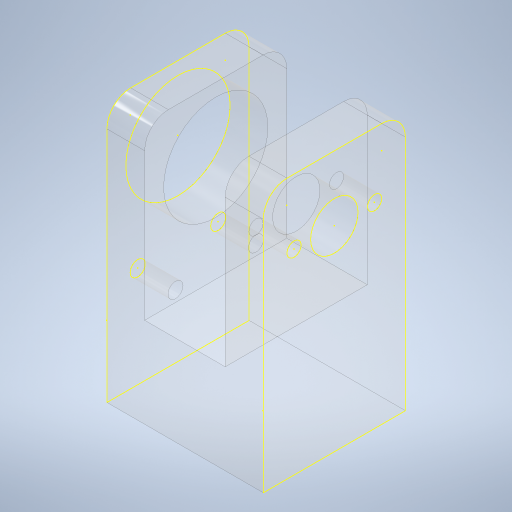
# Autodesk Inventor part: base
Saved by Autodesk Inventor 2024 (Build 280153000, 153)
## iProperties
Created: 2024-08-05
Part Number: base
Material: Polycarbonate, Clear
Document SubType Name: Modeling
Designer: David Ricaurte
Density: 1.2 g/cm^3
Appearance: Polycarbonate - Clear
Mass: 38.4086 g
Surface Area: 98.7251 cm^2
Volume: 32.0072 cm^3
Author: David Ricaurte
Autodesk Inventor part; units mm, degrees
ref_plane "YZ Plane" through (0, 0, 0) normal (1, 0, 0) x (0, 1, 0)
ref_plane "XZ Plane" through (0, 0, 0) normal (0, 1, 0) x (-1, 0, 0)
ref_plane "XY Plane" through (0, 0, 0) normal (0, 0, 1) x (1, 0, 0)
sketch "Sketch1" plane through (0, 0, 0) normal (1, 0, 0) x (0, 1, 0)
  line L0 (0, 0) -> (40, 0)
  line L1 (40, 0) -> (40, -30)
  line L2 (40, -30) -> (0, -30)
  line L3 (0, -30) -> (0, 0)
  line L4 (0, -15) -> (26.2886, -15)
  circle A0 centre (26.2886, -15) radius 8.5
  circle A1 centre (26.2886, -23.5) radius 1.5
  circle A2 centre (26.2886, -6.5) radius 1.5
  circle A3 centre (26.2886, -15) radius 5
  dimension "d0" = 40
  dimension "d1" = 30
  dimension "d2" = 17
  dimension "d3" = 3
  dimension "d4" = 3
  dimension "d5" = 10
  constraints: 10 end point, 4 centre point, 2 coincident, 2 horizontal, 2 parallel, 2 point on circle, 1 midpoint, 1 perpendicular
  measures "d0" distance of L1.end L2.end
  measures "d1" distance of L0.end L1.end
  measures "d2" diameter of A0
  measures "d3" diameter of A1
  measures "d4" diameter of A2
  measures "d5" diameter of A3
extrude "Extrusion1" add sketch "Sketch1" along normal blind 8 contours A0 A2 A1 | L0 L1 L2 L3
sketch "Sketch2" plane through (0, 0, 0) normal (-1, 0, 0) x (0, 0, 1)
  line L0 (0, 40) -> (0, 0) projected
  line L1 (-30, 0) -> (-30, 40) projected
  line L2 (0, 0) -> (-30, 0)
  line L3 (-30, 0) -> (-30, 4)
  line L4 (-30, 4) -> (0, 4)
  line L5 (0, 4) -> (0, 0)
  dimension "d8" = 4
  constraints: 8 end point, 2 parallel, 1 horizontal, 1 perpendicular, 1 point on line
  measures "d8" distance of L2.end L3.end
extrude "Extrusion2" add sketch "Sketch2" along normal blind 17
sketch "Sketch3" plane through (-17, 0, 0) normal (-1, 0, 0) x (0, 0, 1)
  line L0 (0, 40) -> (0, 0) projected
  line L1 (-30, 40) -> (0, 40) projected
  line L2 (0, 0) -> (-30, 0)
  line L3 (-30, 0) -> (-30, 40)
  line L4 (-30, 40) -> (0, 40)
  line L5 (0, 40) -> (0, 0)
  constraints: 8 end point, 2 parallel, 1 horizontal, 1 perpendicular
extrude "Extrusion3" add sketch "Sketch3" along normal blind 8
sketch "Sketch4" plane through (-17, 0, 0) normal (1, 0, 0) x (0, 0, -1)
  circle A0 centre (15, 26.2886) radius 5 projected
  circle A1 centre (15, 26.2886) radius 11
  point P0 (0, 0)
  dimension "d13" = 22
  constraints: 1 centre point, 1 coincident
  measures "d13" diameter of A1
extrude "Extrusion4" cut sketch "Sketch4" against normal through all contours A0 | A1
fillet "Fillet1" radius 5 4 edges at (4, 40, 0) (-21, 40, 0) (-21, 40, -30) (4, 40, -30)
sketch "Sketch5" plane through (-25, 0, 0) normal (-1, 0, 0) x (0, 0, 1)
  circle A0 centre (-15, 26.2886) radius 11 projected
  line L0 (-15, 26.2886) -> (-15, 6.2886)
  line L1 (-15, 6.2886) -> (-6.5, 6.2886)
  line L2 (-30, 35) -> (-30, 4) projected
  line L3 (-6.5, 6.2886) -> (-23.5, 6.2886)
  circle A1 centre (-6.5, 6.2886) radius 1.6
  circle A2 centre (-23.5, 6.2886) radius 1.6
  point P0 (0, 0)
  dimension "d17" = 20
  dimension "d18" = 8.5
  dimension "d19" = 17
  dimension "d20" = 3.2
  dimension "d21" = 3.2
  constraints: 6 end point, 2 centre point, 2 coincident, 1 perpendicular, 1 point on line, 1 vertical
  measures "d17" distance of L0.start L0.end
  measures "d18" distance of L0.end L1.end
  measures "d19" distance of L1.end L3.end
  measures "d20" diameter of A1
  measures "d21" diameter of A2
extrude "Extrusion5" cut sketch "Sketch5" against normal blind 10 contours A1 | A2
sketch "Sketch6" plane through (-25, 0, 0) normal (-1, 0, 0) x (0, 0, 1)
  line L0 (-30, 0) -> (-30, 35) projected
  line L1 (-30, 0) -> (0, 0)
  line L2 (0, 0) -> (0, -15)
  line L3 (0, -15) -> (-30, -15)
  line L4 (-30, -15) -> (-30, 0)
  dimension "d24" = 15
  constraints: 8 end point, 2 parallel, 1 horizontal, 1 perpendicular
  measures "d24" distance of L1.end L2.end
extrude "Extrusion6" add sketch "Sketch6" against normal blind 33
sketch "Sketch7" plane through (8, 0, 0) normal (1, 0, 0) x (0, 0, -1)
  arc A0 (30, 35) -> (25, 40) centre (25, 35) ccw projected
  line L0 (25, 40) -> (5, 40) projected
  arc A1 (5, 40) -> (0, 35) centre (5, 35) ccw projected
  line L1 (0, 35) -> (0, -15) projected
  line L2 (0, -15) -> (30, -15) projected
  line L3 (30, -15) -> (30, 35) projected
  circle A2 centre (23.5, 26.2886) radius 1.5 projected
  circle A3 centre (6.5, 26.2886) radius 1.5 projected
  circle A4 centre (15, 26.2886) radius 5 projected
  point P0 (0, 0)
sketch "Sketch8" plane through (-25, 0, 0) normal (-1, 0, 0) x (0, 0, 1)
  circle A0 centre (-23.5, 6.2886) radius 1.6 projected
  circle A1 centre (-6.5, 6.2886) radius 1.6 projected
  circle A2 centre (-15, 26.2886) radius 11 projected
  arc A3 (-25, 40) -> (-30, 35) centre (-25, 35) ccw projected
  line L0 (-30, 35) -> (-30, -15) projected
  line L1 (-30, -15) -> (0, -15) projected
  line L2 (0, -15) -> (0, 35) projected
  arc A4 (0, 35) -> (-5, 40) centre (-5, 35) ccw projected
  line L3 (-5, 40) -> (-25, 40) projected
  point P0 (0, 0)
body "Solid1"
